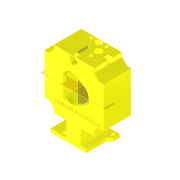
# Autodesk Inventor part: 20_Cube_Insert_Autofocus_KES400a_mirrorinsert
Saved by Autodesk Inventor 2022 (Build 260153000, 153)
## iProperties
Created: 2019-07-01
Part Number: 20_Cube_Insert_Autofocus_KES400a_mirrorinsert
Material: Generic
Document SubType Name: Modeling
Designer: diederichbenedict
Density: 1 g/cm^3
Appearance: Glatt - Gelb
Author: diederichbenedict
Autodesk Inventor part; units mm, degrees
ref_plane "YZ Plane" through (0, 0, 0) normal (1, 0, 0) x (0, 1, 0)
ref_plane "XZ Plane" through (0, 0, 0) normal (0, 1, 0) x (-1, 0, 0)
ref_plane "Work Plane1" through (-56.3599, 0, 22) normal (0, 0, -1) x (-1, 0, 0)
sketch "Sketch1" plane through (-56.3599, 0, 22) normal (0, 0, -1) x (-1, 0, 0)
  line L0 (-4.0299, -0.3538) -> (-2.2322, 1.4439) construction
  arc A0 (-1.4439, 2.2322) -> (-2.2322, 1.4439) centre (-0.9299, 0.9299) ccw construction
  line L1 (-1.4439, 2.2322) -> (0.3538, 4.0299) construction
  line L2 (-37.8299, 42.8299) -> (-37.8299, 37.8299) construction
  line L3 (-37.8299, 37.8299) -> (-42.9208, 37.8299) construction
  line L4 (-37.8299, 42.2137) -> (-37.8299, 45.8299) construction
  line L5 (-37.8299, 45.8299) -> (-4.0299, 45.8299) construction
  line L6 (-4.0299, 45.8299) -> (-4.0299, 42.2137) construction
  line L7 (-4.0299, 4.0299) -> (0.3538, 4.0299) projected
  circle A1 centre (-20.9299, 20.9299) radius 17.5 projected
  line L8 (-20.9299, 58.9723) -> (17.1124, 20.9299) construction
  line L9 (17.1124, 20.9299) -> (-20.9299, -17.1124) construction
  line L10 (-20.9299, -17.1124) -> (-58.9723, 20.9299) construction
  line L11 (-58.9723, 20.9299) -> (-20.9299, 58.9723) construction
  line L12 (-20.9299, 58.9723) -> (-20.9299, -17.1124) construction
  line L13 (17.1124, 20.9299) -> (-58.9723, 20.9299) construction
  line L14 (-20.9299, 58.9723) -> (32.8701, 58.9723) construction
  line L15 (-43.4299, 43.4299) -> (1.5701, 43.4299) construction
  line L16 (1.5701, 43.4299) -> (1.5701, -1.5701) construction
  line L17 (1.5701, -1.5701) -> (-43.4299, -1.5701) construction
  line L18 (-43.4299, -1.5701) -> (-43.4299, 43.4299) construction
  line L19 (-43.4299, 43.4299) -> (1.5701, -1.5701) construction
  line L20 (1.5701, 43.4299) -> (-43.4299, -1.5701) construction
  line L21 (-43.4299, 5.3876) -> (-43.4299, 36.4723)
  line L22 (-43.4299, 36.4723) -> (-36.4723, 43.4299)
  line L23 (-36.4723, 43.4299) -> (-5.3876, 43.4299)
  line L24 (-5.3876, 43.4299) -> (1.5701, 36.4723)
  line L25 (1.5701, 36.4723) -> (1.5701, 5.3876)
  line L26 (1.5701, 5.3876) -> (-5.3876, -1.5701)
  line L27 (-5.3876, -1.5701) -> (-36.4723, -1.5701)
  line L28 (-36.4723, -1.5701) -> (-43.4299, 5.3876)
  line L29 (-4.0299, 42.2137) -> (-37.8299, 42.2137) projected
  line L30 (-4.0299, -0.3538) -> (-4.0299, 4.0299) projected
  circle A2 centre (-20.9299, 20.9299) radius 1.5
  line L31 (-10.9299, 10.9299) -> (-30.9299, 10.9299) construction
  line L32 (-30.9299, 10.9299) -> (-30.9299, 30.9299) construction
  line L33 (-30.9299, 30.9299) -> (-10.9299, 30.9299) construction
  line L34 (-10.9299, 30.9299) -> (-10.9299, 10.9299) construction
  line L35 (-10.9299, 10.9299) -> (-30.9299, 30.9299) construction
  line L36 (-30.9299, 10.9299) -> (-10.9299, 30.9299) construction
  circle A3 centre (-30.9299, 30.9299) radius 1.4
  circle A4 centre (-30.9299, 10.9299) radius 1.4
  circle A5 centre (-10.9299, 10.9299) radius 1.4
  line L37 (-45.8299, 37.8299) -> (-42.0723, 37.8299) construction
  line L38 (-42.1723, 37.7299) -> (-45.8299, 37.7299)
  line L39 (-45.8299, 37.7299) -> (-45.8299, 4.1299)
  line L40 (-45.8299, 4.1299) -> (-42.1723, 4.1299)
  line L41 (-42.1723, 4.1299) -> (-42.1723, 37.7299)
  line L42 (-45.8299, 4.0299) -> (-42.0723, 4.0299) construction
  line L43 (-45.8299, 37.8299) -> (-42.0723, 37.8299) projected
  line L44 (-37.7299, 45.8299) -> (-4.1299, 45.8299)
  line L45 (-4.1299, 45.8299) -> (-4.1299, 42.1723)
  line L46 (-4.1299, 42.1723) -> (-37.7299, 42.1723)
  line L47 (-37.7299, 42.1723) -> (-37.7299, 45.8299)
  line L48 (0.4701, 37.8299) -> (0.4701, 4.0299) construction
  line L49 (0.4701, 4.0299) -> (3.9701, 4.0299) construction
  line L50 (3.9701, 37.8299) -> (3.9701, 4.0299) construction
  line L51 (0.4701, 37.8299) -> (3.9701, 37.8299) construction
  line L52 (-45.8299, -3.9701) -> (-4.0299, -3.9701) construction
  line L53 (0.3124, 37.7299) -> (3.9701, 37.7299)
  line L54 (3.9701, 37.7299) -> (3.9701, 4.1299)
  line L55 (3.9701, 4.1299) -> (0.3124, 4.1299)
  line L56 (0.3124, 4.1299) -> (0.3124, 37.7299)
  line L57 (-4.1299, -0.3538) -> (-37.7299, -0.3538)
  line L58 (-37.7299, -0.3538) -> (-37.7299, -3.9701)
  line L59 (-37.7299, -3.9701) -> (-4.1299, -3.9701)
  line L60 (-4.1299, -3.9701) -> (-4.1299, -0.3538)
  line L61 (-14.9299, -3.9701) -> (-26.9299, -3.9701)
  line L62 (-26.9299, -3.9701) -> (-26.9299, -15.9701)
  line L63 (-26.9299, -15.9701) -> (-14.9299, -15.9701)
  line L64 (-14.9299, -15.9701) -> (-14.9299, -3.9701)
  line L65 (-14.9299, -3.9701) -> (-26.9299, -15.9701) construction
  line L66 (-26.9299, -3.9701) -> (-14.9299, -15.9701) construction
  point P0 (-37.8299, 4.0299)
  point P1 (-20.9299, -9.9701)
  point P2 (-20.9299, -3.9701)
  point P3 (-14.9299, -3.9701)
  point P4 (-4.1713, -0.3538)
  point P5 (0.3124, 4.1299)
  point P6 (-42.1723, 4.1299)
  point P7 (-37.6885, -0.3538)
  point P8 (-26.9299, -3.9701)
  dimension "d18" = 53.8
  dimension "d19" = 45
  dimension "d20" = 53.8
  dimension "d21" = 45
  dimension "d22" = 45
  dimension "d30" = 20
  dimension "d31" = 20
  dimension "d32" = 2.8
  dimension "d33" = 2.8
  dimension "d34" = 2.8
  dimension "d35" = 3
  dimension "d36" = 0.1
  dimension "d37" = 0.1
  dimension "d38" = 0.1
  dimension "d39" = 0.1
  dimension "d196" = 12
  dimension "d197" = 12
  constraints: 98 end point, 22 point on line, 16 parallel, 11 midpoint, 9 perpendicular, 8 horizontal, 4 centre point, 4 coincident, 1 equal length
  measures "d18" distance of L8.start L8.end
  measures "d19" angle of L8 L14
  measures "d20" distance of L8.end L9.end
  measures "d21" distance of L16.end L17.end
  measures "d22" distance of L15.end L16.end
  measures "d30" distance of L32.end L33.end
  measures "d31" distance of L31.end L32.end
  measures "d32" diameter of A3
  measures "d33" diameter of A4
  measures "d34" diameter of A5
  measures "d35" diameter of A2
  measures "d36" distance between parallel lines of L38 L43
  measures "d37" distance between parallel lines of L40 L42
  measures "d38" distance between parallel lines of L45 L6
  measures "d39" distance between parallel lines of L4 L47
  measures "d196" distance of L63.end L62.end
  measures "d197" distance of L62.end L61.end
extrude "Extrusion1" add sketch "Sketch1" along normal blind 24 contours L30 L26 L57 L28 L41 L22 L46 L24 L56 L7 | L7 L26 L30 | L56 L24 L25 L26 | L26 L25 L24 L53 L54 L55 | L57 L60 L59 L58 L28 L27 L26 | L26 L27 L28 L57 | L46 L22 L29 L24 | L24 L29 L45 | L40 L39 L38 L22 L21 L28 | L28 L21 L22 L41 | L29 L22 L23 L24 | L24 L23 L22 L29 L47 L44 L45 | L47 L29 L22 | L64 L63 L62 L59 | A1 | A2 | A3 | A4 | A5
sketch "Skizze4" plane through (-56.3599, 0, -2) normal (0, 0, -1) x (-1, 0, 0)
  line L0 (-37.7299, 42.1723) -> (-42.1723, 37.7299) projected
  line L1 (-42.1723, 37.7299) -> (-45.8299, 37.7299) projected
  line L2 (-45.8299, 37.7299) -> (-45.8299, 4.1299) construction
  line L3 (-45.8299, 4.1299) -> (-42.1723, 4.1299) projected
  line L4 (-42.1723, 4.1299) -> (-37.6885, -0.3538) projected
  line L5 (-37.6885, -0.3538) -> (-37.7299, -0.3538) projected
  line L6 (-37.7299, -0.3538) -> (-37.7299, -3.9701) projected
  line L7 (-37.7299, -3.9701) -> (-26.9299, -3.9701) construction
  line L8 (-4.1299, -3.9701) -> (-4.1299, -0.3538) projected
  line L9 (-4.1713, -0.3538) -> (0.3124, 4.1299) projected
  line L10 (0.3124, 4.1299) -> (3.9701, 4.1299) projected
  line L11 (3.9701, 4.1299) -> (3.9701, 37.7299) construction
  line L12 (3.9701, 37.7299) -> (0.3124, 37.7299) projected
  line L13 (0.3124, 37.7299) -> (-4.1299, 42.1723) projected
  line L14 (-4.1299, 42.1723) -> (-4.1299, 45.8299) projected
  line L15 (-4.1299, 45.8299) -> (-37.7299, 45.8299) construction
  line L16 (-37.7299, 45.8299) -> (-37.7299, 42.1723) projected
  line L17 (-37.9299, 46.0299) -> (-3.9299, 46.0299) construction
  line L18 (-3.9299, 46.0299) -> (-3.9299, 42.2551)
  line L19 (-3.9299, 42.2551) -> (0.3953, 37.9299)
  line L20 (0.3953, 37.9299) -> (4.1701, 37.9299)
  line L21 (4.1701, 37.9299) -> (4.1701, 3.9299) construction
  line L22 (4.1701, 3.9299) -> (0.3953, 3.9299)
  line L23 (0.3953, 3.9299) -> (-3.9299, -0.3953)
  line L24 (-3.9299, -0.3953) -> (-3.9299, -4.1701)
  line L25 (-3.9299, -4.1701) -> (-37.9299, -4.1701) construction
  line L26 (-37.9299, -4.1701) -> (-37.9299, -0.3953)
  line L27 (-37.9299, -0.3953) -> (-42.2551, 3.9299)
  line L28 (-42.2551, 3.9299) -> (-46.0299, 3.9299)
  line L29 (-46.0299, 3.9299) -> (-46.0299, 37.9299) construction
  line L30 (-46.0299, 37.9299) -> (-42.2551, 37.9299)
  line L31 (-42.2551, 37.9299) -> (-37.9299, 42.2551)
  line L32 (-37.9299, 42.2551) -> (-37.9299, 46.0299)
  line L33 (-45.8299, 37.7299) -> (-45.8299, 37.9299)
  line L34 (-4.1299, 45.8299) -> (-37.7299, 45.8299) projected
  line L35 (-37.7299, 45.8299) -> (-37.9299, 45.8299)
  line L36 (-4.1299, 45.8299) -> (-3.9299, 45.8299)
  line L37 (3.9701, 37.7299) -> (3.9701, 37.9299)
  line L38 (3.9701, 4.1299) -> (3.9701, 37.7299) projected
  line L39 (3.9701, 4.1299) -> (3.9701, 3.9299)
  line L40 (-4.1299, -3.9701) -> (-3.9299, -3.9701)
  line L41 (-37.7299, -3.9701) -> (-37.9299, -3.9701)
  line L42 (-45.8299, 4.1299) -> (-45.8299, 3.9299)
  line L43 (-4.1299, -0.3538) -> (-4.1713, -0.3538) projected
  line L44 (-14.9299, -15.9701) -> (-14.9299, -3.9701) projected
  line L45 (-14.9299, -3.9701) -> (-4.1299, -3.9701) projected
  line L46 (-26.9299, -3.9701) -> (-26.9299, -15.9701) projected
  line L47 (-26.9299, -15.9701) -> (-14.9299, -15.9701) projected
  point P0 (-56.3599, 0)
  dimension "d40" = 0.2
  constraints: 48 end point, 12 point on line, 4 perpendicular, 15 other
  measures "d40" distance between parallel lines of L15 L17
extrude "IM_offset" add sketch "Skizze4" against normal up to surface (24 mm away)
ref_plane "Arbeitsebene5" through (-35.4299, 3.9299, 22) normal (-1, 0, 0) x (0, 0, 1)
ref_plane "Arbeitsebene6" through (-18.4299, 20.9299, 22) normal (0, 1, 0) x (-1, 0, 0)
chamfer "Fase2" distance 0.5 angle 45 34 edges at (-35.4299, 45.8299, 22) (-18.4299, 44.0425, 22) (-16.2673, 40.0925, 22) (-12.3173, 37.9299, 22) (-10.5299, 20.9299, 22) (-12.3173, 3.9299, 22) (-16.2673, 1.7673, 22) (-18.4299, -2.1827, 22) (-46.9299, -3.9701, 22) (-23.9299, -3.9701, 22) (-52.4299, -2.1827, 22) (-54.5925, 1.7673, 22) (-58.5425, 3.9299, 22) (-60.3299, 20.9299, 22) (-58.5425, 37.9299, 22) (-54.5925, 40.0925, 22) (-54.5925, 1.7673, -2) (-58.5425, 3.9299, -2) (-60.3299, 20.9299, -2) (-52.4299, -2.1827, -2) (-46.9299, -3.9701, -2) (-23.9299, -3.9701, -2) (-18.4299, -2.1827, -2) (-16.2673, 1.7673, -2) (-12.3173, 3.9299, -2) (-10.5299, 20.9299, -2) (-12.3173, 37.9299, -2) (-16.2673, 40.0925, -2) (-18.4299, 44.0425, -2) (-35.4299, 45.8299, -2) (-52.4299, 44.0425, -2) (-54.5925, 40.0925, -2) (-58.5425, 37.9299, -2) (-52.4299, 44.0425, 22)
sketch "Skizze32" plane through (-56.3599, 0, 22) normal (0, 0, 1) x (1, 0, 0)
  line L0 (4.6074, 8.4523) -> (68.202, 8.4523) construction
  line L1 (68.202, 8.4523) -> (68.202, -1.1922) construction
  line L2 (68.202, -1.1922) -> (4.6074, -1.1922) construction
  line L3 (4.6074, -1.1922) -> (4.6074, 8.4523) construction
  line L4 (7.5956, 5.2466) -> (6.6687, 5.2466)
  line L5 (6.6687, 5.2466) -> (5.8407, 6.4848)
  line L6 (5.8407, 6.4848) -> (5.69, 6.2772)
  line L7 (5.69, 6.2772) -> (5.69, 5.2466)
  line L8 (5.69, 5.2466) -> (4.9237, 5.2466)
  line L9 (4.9237, 5.2466) -> (4.9237, 8.2966)
  line L10 (4.9237, 8.2966) -> (5.69, 8.2966)
  line L11 (5.69, 8.2966) -> (5.69, 6.9347)
  line L12 (5.69, 6.9347) -> (6.6687, 8.2966)
  line L13 (6.6687, 8.2966) -> (7.5511, 8.2966)
  line L14 (7.5511, 8.2966) -> (6.4636, 6.8803)
  line L15 (6.4636, 6.8803) -> (7.5956, 5.2466)
  line L16 (7.8452, 5.2466) -> (7.8452, 8.2966)
  line L17 (7.8452, 8.2966) -> (9.9066, 8.2966)
  line L18 (9.9066, 8.2966) -> (9.9066, 7.7157)
  line L19 (9.9066, 7.7157) -> (8.6065, 7.7157)
  line L20 (8.6065, 7.7157) -> (8.6065, 7.1794)
  line L21 (8.6065, 7.1794) -> (9.8052, 7.1794)
  line L22 (9.8052, 7.1794) -> (9.8052, 6.5985)
  line L23 (9.8052, 6.5985) -> (8.6065, 6.5985)
  line L24 (8.6065, 6.5985) -> (8.6065, 5.8274)
  line L25 (8.6065, 5.8274) -> (9.9066, 5.8274)
  line L26 (9.9066, 5.8274) -> (9.9066, 5.2466)
  line L27 (9.9066, 5.2466) -> (7.8452, 5.2466)
  spline S0 degree 2 poles (11.3673, 5.1922) (11.0163, 5.1922) (10.4874, 5.3281) (10.26, 5.427) knots 0 0 0 1 2 2 2
  line L28 (10.26, 5.427) -> (10.26, 6.1536)
  line L29 (10.26, 6.1536) -> (10.3292, 6.1536)
  spline S1 degree 2 poles (10.3292, 6.1536) (10.5591, 5.9584) (11.1103, 5.7483) (11.3698, 5.7483) knots 0 0 0 1 2 2 2
  spline S2 degree 2 poles (11.3698, 5.7483) (11.4365, 5.7483) (11.6515, 5.778) (11.7158, 5.8076) knots 0 0 0 1 2 2 2
  spline S3 degree 2 poles (11.7158, 5.8076) (11.7949, 5.8422) (11.9061, 5.9683) (11.9061, 6.0696) knots 0 0 0 1 2 2 2
  spline S4 degree 2 poles (11.9061, 6.0696) (11.9061, 6.1858) (11.7257, 6.3291) (11.6021, 6.3613) knots 0 0 0 1 2 2 2
  spline S5 degree 2 poles (11.6021, 6.3613) (11.4464, 6.4033) (11.093, 6.475) (10.9372, 6.5293) knots 0 0 0 1 2 2 2
  spline S6 degree 2 poles (10.9372, 6.5293) (10.5838, 6.6529) (10.2773, 7.0756) (10.2773, 7.3919) knots 0 0 0 1 2 2 2
  spline S7 degree 2 poles (10.2773, 7.3919) (10.2773, 7.8195) (11.0015, 8.3509) (11.5453, 8.3509) knots 0 0 0 1 2 2 2
  spline S8 degree 2 poles (11.5453, 8.3509) (11.8171, 8.3509) (12.356, 8.2397) (12.5685, 8.1458) knots 0 0 0 1 2 2 2
  line L30 (12.5685, 8.1458) -> (12.5685, 7.4488)
  line L31 (12.5685, 7.4488) -> (12.5018, 7.4488)
  spline S9 degree 2 poles (12.5018, 7.4488) (12.3312, 7.5946) (11.8419, 7.7948) (11.5848, 7.7948) knots 0 0 0 1 2 2 2
  spline S10 degree 2 poles (11.5848, 7.7948) (11.4835, 7.7948) (11.3253, 7.7652) (11.2363, 7.7256) knots 0 0 0 1 2 2 2
  spline S11 degree 2 poles (11.2363, 7.7256) (11.1646, 7.6935) (11.0608, 7.5649) (11.0608, 7.4859) knots 0 0 0 1 2 2 2
  spline S12 degree 2 poles (11.0608, 7.4859) (11.0608, 7.3672) (11.2264, 7.2313) (11.4637, 7.1769) knots 0 0 0 1 2 2 2
  spline S13 degree 2 poles (11.4637, 7.1769) (11.6169, 7.1423) (11.9012, 7.0756) (12.0643, 7.0187) knots 0 0 0 1 2 2 2
  spline S14 degree 2 poles (12.0643, 7.0187) (12.3807, 6.9025) (12.6896, 6.517) (12.6896, 6.2006) knots 0 0 0 1 2 2 2
  spline S15 degree 2 poles (12.6896, 6.2006) (12.6896, 5.7458) (11.9753, 5.1922) (11.3673, 5.1922) knots 0 0 0 1 2 2 2
  line L32 (15.3541, 5.9584) -> (14.9413, 5.9584)
  line L33 (14.9413, 5.9584) -> (14.9413, 5.2391)
  line L34 (14.9413, 5.2391) -> (14.2023, 5.2391)
  line L35 (14.2023, 5.2391) -> (14.2023, 5.9584)
  line L36 (14.2023, 5.9584) -> (12.8577, 5.9584)
  line L37 (12.8577, 5.9584) -> (12.8577, 6.5269)
  line L38 (12.8577, 6.5269) -> (14.1776, 8.2966)
  line L39 (14.1776, 8.2966) -> (14.9413, 8.2966)
  line L40 (14.9413, 8.2966) -> (14.9413, 6.5071)
  line L41 (14.9413, 6.5071) -> (15.3541, 6.5071)
  line L42 (15.3541, 6.5071) -> (15.3541, 5.9584)
  line L43 (14.2023, 6.5071) -> (14.2023, 7.5452)
  line L44 (14.2023, 7.5452) -> (13.4287, 6.5071)
  line L45 (13.4287, 6.5071) -> (14.2023, 6.5071)
  spline S16 degree 2 poles (17.9493, 6.7716) (17.9493, 6.3761) (17.8232, 5.7829) (17.6823, 5.5827) knots 0 0 0 1 2 2 2
  spline S17 degree 2 poles (17.6823, 5.5827) (17.5439, 5.385) (17.0966, 5.1823) (16.7752, 5.1823) knots 0 0 0 1 2 2 2
  spline S18 degree 2 poles (16.7752, 5.1823) (16.4515, 5.1823) (16.0066, 5.385) (15.8657, 5.5876) knots 0 0 0 1 2 2 2
  spline S19 degree 2 poles (15.8657, 5.5876) (15.7248, 5.7878) (15.5987, 6.3761) (15.5987, 6.7716) knots 0 0 0 1 2 2 2
  spline S20 degree 2 poles (15.5987, 6.7716) (15.5987, 7.1769) (15.7248, 7.7503) (15.8682, 7.9579) knots 0 0 0 1 2 2 2
  spline S21 degree 2 poles (15.8682, 7.9579) (16.0115, 8.1606) (16.4638, 8.3583) (16.7752, 8.3583) knots 0 0 0 1 2 2 2
  spline S22 degree 2 poles (16.7752, 8.3583) (17.104, 8.3583) (17.5439, 8.1507) (17.6848, 7.9456) knots 0 0 0 1 2 2 2
  spline S23 degree 2 poles (17.6848, 7.9456) (17.8232, 7.7454) (17.9493, 7.1547) (17.9493, 6.7716) knots 0 0 0 1 2 2 2
  spline S24 degree 2 poles (17.1806, 6.7716) (17.1806, 7.3376) (16.9952, 7.7948) (16.7752, 7.7948) knots 0 0 0 1 2 2 2
  spline S25 degree 2 poles (16.7752, 7.7948) (16.5553, 7.7948) (16.3674, 7.3376) (16.3674, 6.7691) knots 0 0 0 1 2 2 2
  spline S26 degree 2 poles (16.3674, 6.7691) (16.3674, 6.2105) (16.5553, 5.7458) (16.7752, 5.7458) knots 0 0 0 1 2 2 2
  spline S27 degree 2 poles (16.7752, 5.7458) (16.9928, 5.7458) (17.1806, 6.2105) (17.1806, 6.7716) knots 0 0 0 1 2 2 2
  spline S28 degree 2 poles (20.6211, 6.7716) (20.6211, 6.3761) (20.4951, 5.7829) (20.3542, 5.5827) knots 0 0 0 1 2 2 2
  spline S29 degree 2 poles (20.3542, 5.5827) (20.2158, 5.385) (19.7684, 5.1823) (19.4471, 5.1823) knots 0 0 0 1 2 2 2
  spline S30 degree 2 poles (19.4471, 5.1823) (19.1233, 5.1823) (18.6784, 5.385) (18.5375, 5.5876) knots 0 0 0 1 2 2 2
  spline S31 degree 2 poles (18.5375, 5.5876) (18.3966, 5.7878) (18.2706, 6.3761) (18.2706, 6.7716) knots 0 0 0 1 2 2 2
  spline S32 degree 2 poles (18.2706, 6.7716) (18.2706, 7.1769) (18.3966, 7.7503) (18.54, 7.9579) knots 0 0 0 1 2 2 2
  spline S33 degree 2 poles (18.54, 7.9579) (18.6834, 8.1606) (19.1357, 8.3583) (19.4471, 8.3583) knots 0 0 0 1 2 2 2
  spline S34 degree 2 poles (19.4471, 8.3583) (19.7758, 8.3583) (20.2158, 8.1507) (20.3566, 7.9456) knots 0 0 0 1 2 2 2
  spline S35 degree 2 poles (20.3566, 7.9456) (20.4951, 7.7454) (20.6211, 7.1547) (20.6211, 6.7716) knots 0 0 0 1 2 2 2
  spline S36 degree 2 poles (19.8524, 6.7716) (19.8524, 7.3376) (19.6671, 7.7948) (19.4471, 7.7948) knots 0 0 0 1 2 2 2
  spline S37 degree 2 poles (19.4471, 7.7948) (19.2271, 7.7948) (19.0393, 7.3376) (19.0393, 6.7691) knots 0 0 0 1 2 2 2
  spline S38 degree 2 poles (19.0393, 6.7691) (19.0393, 6.2105) (19.2271, 5.7458) (19.4471, 5.7458) knots 0 0 0 1 2 2 2
  spline S39 degree 2 poles (19.4471, 5.7458) (19.6646, 5.7458) (19.8524, 6.2105) (19.8524, 6.7716) knots 0 0 0 1 2 2 2
  line L46 (21.9978, 5.2466) -> (23.0285, 8.2966)
  line L47 (23.0285, 8.2966) -> (23.8639, 8.2966)
  line L48 (23.8639, 8.2966) -> (24.8946, 5.2466)
  line L49 (24.8946, 5.2466) -> (24.1061, 5.2466)
  line L50 (24.1061, 5.2466) -> (23.9158, 5.8694)
  line L51 (23.9158, 5.8694) -> (22.9568, 5.8694)
  line L52 (22.9568, 5.8694) -> (22.764, 5.2466)
  line L53 (22.764, 5.2466) -> (21.9978, 5.2466)
  line L54 (23.7477, 6.4231) -> (23.4363, 7.4315)
  line L55 (23.4363, 7.4315) -> (23.1224, 6.4231)
  line L56 (23.1224, 6.4231) -> (23.7477, 6.4231)
  line L57 (27.2921, 5.2466) -> (26.5753, 5.2466)
  line L58 (26.5753, 5.2466) -> (26.5753, 5.5011)
  spline S40 degree 2 poles (26.5753, 5.5011) (26.3899, 5.3454) (26.0785, 5.1823) (25.8635, 5.1823) knots 0 0 0 1 2 2 2
  spline S41 degree 2 poles (25.8635, 5.1823) (25.5224, 5.1823) (25.1393, 5.6148) (25.1393, 6.0498) knots 0 0 0 1 2 2 2
  line L59 (25.1393, 6.0498) -> (25.1393, 7.5476)
  line L60 (25.1393, 7.5476) -> (25.861, 7.5476)
  line L61 (25.861, 7.5476) -> (25.861, 6.4058)
  spline S42 degree 2 poles (25.861, 6.4058) (25.861, 6.2278) (25.8783, 6.0004) (25.9129, 5.9238) knots 0 0 0 1 2 2 2
  spline S43 degree 2 poles (25.9129, 5.9238) (25.9475, 5.8521) (26.0834, 5.778) (26.207, 5.778) knots 0 0 0 1 2 2 2
  spline S44 degree 2 poles (26.207, 5.778) (26.2812, 5.778) (26.4888, 5.8521) (26.5753, 5.9164) knots 0 0 0 1 2 2 2
  line L62 (26.5753, 5.9164) -> (26.5753, 7.5476)
  line L63 (26.5753, 7.5476) -> (27.2921, 7.5476)
  line L64 (27.2921, 7.5476) -> (27.2921, 5.2466)
  spline S45 degree 2 poles (28.7207, 5.2021) (28.2832, 5.2021) (27.8828, 5.5629) (27.8828, 5.9732) knots 0 0 0 1 2 2 2
  line L65 (27.8828, 5.9732) -> (27.8828, 7.0484)
  line L66 (27.8828, 7.0484) -> (27.6084, 7.0484)
  line L67 (27.6084, 7.0484) -> (27.6084, 7.5476)
  line L68 (27.6084, 7.5476) -> (27.8828, 7.5476)
  line L69 (27.8828, 7.5476) -> (27.8828, 8.2051)
  line L70 (27.8828, 8.2051) -> (28.5996, 8.2051)
  line L71 (28.5996, 8.2051) -> (28.5996, 7.5476)
  line L72 (28.5996, 7.5476) -> (29.2916, 7.5476)
  line L73 (29.2916, 7.5476) -> (29.2916, 7.0484)
  line L74 (29.2916, 7.0484) -> (28.5996, 7.0484)
  line L75 (28.5996, 7.0484) -> (28.5996, 6.2303)
  spline S46 degree 2 poles (28.5996, 6.2303) (28.5996, 6.1092) (28.6045, 5.9287) (28.6342, 5.857) knots 0 0 0 1 2 2 2
  spline S47 degree 2 poles (28.6342, 5.857) (28.6638, 5.7854) (28.8096, 5.7013) (28.9481, 5.7013) knots 0 0 0 1 2 2 2
  spline S48 degree 2 poles (28.9481, 5.7013) (29.0074, 5.7013) (29.1928, 5.7508) (29.2298, 5.7705) knots 0 0 0 1 2 2 2
  line L76 (29.2298, 5.7705) -> (29.2916, 5.7705)
  line L77 (29.2916, 5.7705) -> (29.2916, 5.2663)
  spline S49 degree 2 poles (29.2916, 5.2663) (29.1754, 5.2367) (28.9135, 5.2021) (28.7207, 5.2021) knots 0 0 0 1 2 2 2
  spline S50 degree 2 poles (31.7904, 6.3959) (31.7904, 5.8274) (31.1701, 5.1749) (30.6041, 5.1749) knots 0 0 0 1 2 2 2
  spline S51 degree 2 poles (30.6041, 5.1749) (30.0405, 5.1749) (29.4152, 5.8274) (29.4152, 6.3959) knots 0 0 0 1 2 2 2
  spline S52 degree 2 poles (29.4152, 6.3959) (29.4152, 6.9693) (30.0405, 7.6193) (30.6041, 7.6193) knots 0 0 0 1 2 2 2
  spline S53 degree 2 poles (30.6041, 7.6193) (31.1676, 7.6193) (31.7904, 6.9668) (31.7904, 6.3959) knots 0 0 0 1 2 2 2
  spline S54 degree 2 poles (31.0564, 6.3909) (31.0564, 6.5961) (30.9896, 6.8704) (30.9303, 6.952) knots 0 0 0 1 2 2 2
  spline S55 degree 2 poles (30.9303, 6.952) (30.866, 7.0385) (30.7054, 7.1052) (30.6041, 7.1052) knots 0 0 0 1 2 2 2
  spline S56 degree 2 poles (30.6041, 7.1052) (30.5052, 7.1052) (30.3495, 7.0459) (30.2852, 6.9619) knots 0 0 0 1 2 2 2
  spline S57 degree 2 poles (30.2852, 6.9619) (30.2234, 6.8828) (30.1493, 6.6035) (30.1493, 6.3909) knots 0 0 0 1 2 2 2
  spline S58 degree 2 poles (30.1493, 6.3909) (30.1493, 6.1808) (30.2185, 5.9213) (30.2753, 5.8422) knots 0 0 0 1 2 2 2
  spline S59 degree 2 poles (30.2753, 5.8422) (30.3322, 5.7631) (30.5052, 5.689) (30.609, 5.689) knots 0 0 0 1 2 2 2
  spline S60 degree 2 poles (30.609, 5.689) (30.6955, 5.689) (30.8735, 5.7631) (30.9278, 5.8373) knots 0 0 0 1 2 2 2
  spline S61 degree 2 poles (30.9278, 5.8373) (30.9896, 5.9238) (31.0564, 6.1734) (31.0564, 6.3909) knots 0 0 0 1 2 2 2
  line L78 (33.6417, 7.8912) -> (33.5873, 7.8912)
  spline S62 degree 2 poles (33.5873, 7.8912) (33.5453, 7.9036) (33.3698, 7.9431) (33.2932, 7.9431) knots 0 0 0 1 2 2 2
  spline S63 degree 2 poles (33.2932, 7.9431) (33.0757, 7.9431) (32.9175, 7.7849) (32.9175, 7.5649) knots 0 0 0 1 2 2 2
  line L79 (32.9175, 7.5649) -> (32.9175, 7.5476)
  line L80 (32.9175, 7.5476) -> (33.4885, 7.5476)
  line L81 (33.4885, 7.5476) -> (33.4885, 7.0484)
  line L82 (33.4885, 7.0484) -> (32.9422, 7.0484)
  line L83 (32.9422, 7.0484) -> (32.9422, 5.2466)
  line L84 (32.9422, 5.2466) -> (32.2254, 5.2466)
  line L85 (32.2254, 5.2466) -> (32.2254, 7.0484)
  line L86 (32.2254, 7.0484) -> (31.9387, 7.0484)
  line L87 (31.9387, 7.0484) -> (31.9387, 7.5476)
  line L88 (31.9387, 7.5476) -> (32.2254, 7.5476)
  line L89 (32.2254, 7.5476) -> (32.2254, 7.6119)
  spline S64 degree 2 poles (32.2254, 7.6119) (32.2254, 8.0321) (32.6679, 8.4523) (33.1177, 8.4523) knots 0 0 0 1 2 2 2
  spline S65 degree 2 poles (33.1177, 8.4523) (33.2734, 8.4523) (33.5428, 8.43) (33.6417, 8.4102) knots 0 0 0 1 2 2 2
  line L90 (33.6417, 8.4102) -> (33.6417, 7.8912)
  spline S66 degree 2 poles (35.9823, 6.3959) (35.9823, 5.8274) (35.362, 5.1749) (34.796, 5.1749) knots 0 0 0 1 2 2 2
  spline S67 degree 2 poles (34.796, 5.1749) (34.2324, 5.1749) (33.6071, 5.8274) (33.6071, 6.3959) knots 0 0 0 1 2 2 2
  spline S68 degree 2 poles (33.6071, 6.3959) (33.6071, 6.9693) (34.2324, 7.6193) (34.796, 7.6193) knots 0 0 0 1 2 2 2
  spline S69 degree 2 poles (34.796, 7.6193) (35.3595, 7.6193) (35.9823, 6.9668) (35.9823, 6.3959) knots 0 0 0 1 2 2 2
  spline S70 degree 2 poles (35.2483, 6.3909) (35.2483, 6.5961) (35.1815, 6.8704) (35.1222, 6.952) knots 0 0 0 1 2 2 2
  spline S71 degree 2 poles (35.1222, 6.952) (35.0579, 7.0385) (34.8973, 7.1052) (34.796, 7.1052) knots 0 0 0 1 2 2 2
  spline S72 degree 2 poles (34.796, 7.1052) (34.6971, 7.1052) (34.5414, 7.0459) (34.4771, 6.9619) knots 0 0 0 1 2 2 2
  spline S73 degree 2 poles (34.4771, 6.9619) (34.4153, 6.8828) (34.3412, 6.6035) (34.3412, 6.3909) knots 0 0 0 1 2 2 2
  spline S74 degree 2 poles (34.3412, 6.3909) (34.3412, 6.1808) (34.4104, 5.9213) (34.4672, 5.8422) knots 0 0 0 1 2 2 2
  spline S75 degree 2 poles (34.4672, 5.8422) (34.5241, 5.7631) (34.6971, 5.689) (34.8009, 5.689) knots 0 0 0 1 2 2 2
  spline S76 degree 2 poles (34.8009, 5.689) (34.8874, 5.689) (35.0654, 5.7631) (35.1197, 5.8373) knots 0 0 0 1 2 2 2
  spline S77 degree 2 poles (35.1197, 5.8373) (35.1815, 5.9238) (35.2483, 6.1734) (35.2483, 6.3909) knots 0 0 0 1 2 2 2
  spline S78 degree 2 poles (37.49, 5.1848) (37.2058, 5.1848) (36.7337, 5.3281) (36.5582, 5.4764) knots 0 0 0 1 2 2 2
  spline S79 degree 2 poles (36.5582, 5.4764) (36.3877, 5.6272) (36.1949, 6.0795) (36.1949, 6.386) knots 0 0 0 1 2 2 2
  spline S80 degree 2 poles (36.1949, 6.386) (36.1949, 6.7172) (36.4025, 7.1794) (36.5829, 7.3277) knots 0 0 0 1 2 2 2
  spline S81 degree 2 poles (36.5829, 7.3277) (36.7535, 7.471) (37.2182, 7.6094) (37.4703, 7.6094) knots 0 0 0 1 2 2 2
  spline S82 degree 2 poles (37.4703, 7.6094) (37.6606, 7.6094) (38.0412, 7.5205) (38.234, 7.4241) knots 0 0 0 1 2 2 2
  line L91 (38.234, 7.4241) -> (38.234, 6.8111)
  line L92 (38.234, 6.8111) -> (38.1425, 6.8111)
  spline S83 degree 2 poles (38.1425, 6.8111) (38.0981, 6.8531) (37.9745, 6.952) (37.9003, 6.9915) knots 0 0 0 1 2 2 2
  spline S84 degree 2 poles (37.9003, 6.9915) (37.8212, 7.036) (37.626, 7.0953) (37.5049, 7.0953) knots 0 0 0 1 2 2 2
  spline S85 degree 2 poles (37.5049, 7.0953) (37.2305, 7.0953) (36.929, 6.7122) (36.929, 6.386) knots 0 0 0 1 2 2 2
  spline S86 degree 2 poles (36.929, 6.386) (36.929, 6.0399) (37.2503, 5.6989) (37.5172, 5.6989) knots 0 0 0 1 2 2 2
  spline S87 degree 2 poles (37.5172, 5.6989) (37.6532, 5.6989) (37.8558, 5.7607) (37.93, 5.8051) knots 0 0 0 1 2 2 2
  spline S88 degree 2 poles (37.93, 5.8051) (38.0017, 5.8472) (38.1055, 5.9411) (38.1425, 5.9782) knots 0 0 0 1 2 2 2
  line L93 (38.1425, 5.9782) -> (38.234, 5.9782)
  line L94 (38.234, 5.9782) -> (38.234, 5.3627)
  spline S89 degree 2 poles (38.234, 5.3627) (38.1722, 5.3355) (38.0116, 5.2663) (37.9275, 5.2441) knots 0 0 0 1 2 2 2
  spline S90 degree 2 poles (37.9275, 5.2441) (37.8237, 5.2144) (37.6408, 5.1848) (37.49, 5.1848) knots 0 0 0 1 2 2 2
  line L95 (40.7106, 5.2466) -> (39.9938, 5.2466)
  line L96 (39.9938, 5.2466) -> (39.9938, 5.5011)
  spline S91 degree 2 poles (39.9938, 5.5011) (39.8084, 5.3454) (39.497, 5.1823) (39.282, 5.1823) knots 0 0 0 1 2 2 2
  spline S92 degree 2 poles (39.282, 5.1823) (38.9409, 5.1823) (38.5578, 5.6148) (38.5578, 6.0498) knots 0 0 0 1 2 2 2
  line L97 (38.5578, 6.0498) -> (38.5578, 7.5476)
  line L98 (38.5578, 7.5476) -> (39.2795, 7.5476)
  line L99 (39.2795, 7.5476) -> (39.2795, 6.4058)
  spline S93 degree 2 poles (39.2795, 6.4058) (39.2795, 6.2278) (39.2968, 6.0004) (39.3314, 5.9238) knots 0 0 0 1 2 2 2
  spline S94 degree 2 poles (39.3314, 5.9238) (39.366, 5.8521) (39.5019, 5.778) (39.6255, 5.778) knots 0 0 0 1 2 2 2
  spline S95 degree 2 poles (39.6255, 5.778) (39.6997, 5.778) (39.9073, 5.8521) (39.9938, 5.9164) knots 0 0 0 1 2 2 2
  line L100 (39.9938, 5.9164) -> (39.9938, 7.5476)
  line L101 (39.9938, 7.5476) -> (40.7106, 7.5476)
  line L102 (40.7106, 7.5476) -> (40.7106, 5.2466)
  spline S96 degree 2 poles (41.9588, 5.1848) (41.7066, 5.1848) (41.2543, 5.296) (41.106, 5.3701) knots 0 0 0 1 2 2 2
  line L103 (41.106, 5.3701) -> (41.106, 5.9757)
  line L104 (41.106, 5.9757) -> (41.1654, 5.9757)
  spline S97 degree 2 poles (41.1654, 5.9757) (41.2173, 5.9361) (41.3483, 5.8422) (41.4644, 5.7903) knots 0 0 0 1 2 2 2
  spline S98 degree 2 poles (41.4644, 5.7903) (41.5658, 5.7434) (41.8154, 5.6766) (41.9637, 5.6766) knots 0 0 0 1 2 2 2
  spline S99 degree 2 poles (41.9637, 5.6766) (42.1145, 5.6766) (42.3468, 5.7705) (42.3468, 5.8719) knots 0 0 0 1 2 2 2
  spline S100 degree 2 poles (42.3468, 5.8719) (42.3468, 5.951) (42.2405, 6.035) (42.0873, 6.0696) knots 0 0 0 1 2 2 2
  spline S101 degree 2 poles (42.0873, 6.0696) (42.0057, 6.0919) (41.7561, 6.1388) (41.6597, 6.1685) knots 0 0 0 1 2 2 2
  spline S102 degree 2 poles (41.6597, 6.1685) (41.3878, 6.2525) (41.1159, 6.5812) (41.1159, 6.8506) knots 0 0 0 1 2 2 2
  spline S103 degree 2 poles (41.1159, 6.8506) (41.1159, 7.0039) (41.2568, 7.2758) (41.3952, 7.382) knots 0 0 0 1 2 2 2
  spline S104 degree 2 poles (41.3952, 7.382) (41.5312, 7.4859) (41.934, 7.6094) (42.1886, 7.6094) knots 0 0 0 1 2 2 2
  spline S105 degree 2 poles (42.1886, 7.6094) (42.4308, 7.6094) (42.8362, 7.513) (42.9746, 7.4463) knots 0 0 0 1 2 2 2
  line L105 (42.9746, 7.4463) -> (42.9746, 6.863)
  line L106 (42.9746, 6.863) -> (42.9178, 6.863)
  spline S106 degree 2 poles (42.9178, 6.863) (42.8807, 6.8927) (42.72, 6.9891) (42.6459, 7.0237) knots 0 0 0 1 2 2 2
  spline S107 degree 2 poles (42.6459, 7.0237) (42.5544, 7.0632) (42.332, 7.1176) (42.2158, 7.1176) knots 0 0 0 1 2 2 2
  spline S108 degree 2 poles (42.2158, 7.1176) (42.0601, 7.1176) (41.8451, 7.0113) (41.8451, 6.9248) knots 0 0 0 1 2 2 2
  spline S109 degree 2 poles (41.8451, 6.9248) (41.8451, 6.8457) (41.9513, 6.7567) (42.1293, 6.7122) knots 0 0 0 1 2 2 2
  spline S110 degree 2 poles (42.1293, 6.7122) (42.2207, 6.69) (42.4605, 6.648) (42.5717, 6.6109) knots 0 0 0 1 2 2 2
  spline S111 degree 2 poles (42.5717, 6.6109) (42.8189, 6.5318) (43.0759, 6.2228) (43.0759, 5.9658) knots 0 0 0 1 2 2 2
  spline S112 degree 2 poles (43.0759, 5.9658) (43.0759, 5.8051) (42.9252, 5.511) (42.7843, 5.4122) knots 0 0 0 1 2 2 2
  spline S113 degree 2 poles (42.7843, 5.4122) (42.6385, 5.3034) (42.2381, 5.1848) (41.9588, 5.1848) knots 0 0 0 1 2 2 2
  point P0 (56.3599, 0)
  constraints: 2 other
extrude "Extrusion27" cut sketch "Skizze32" against normal blind 1
sketch "Skizze33" plane through (-56.3599, 0, 22) normal (0, 0, 1) x (1, 0, 0)
  line L0 (37.4299, -3.4701) -> (26.9299, -3.4701) projected
  line L1 (37.4299, -0.1882) -> (37.4299, -3.4701) projected
  line L2 (42.048, 4.4299) -> (37.4299, -0.1882) projected
  line L3 (45.3299, 4.4299) -> (42.048, 4.4299) projected
  line L4 (45.3299, 37.4299) -> (45.3299, 4.4299) projected
  line L5 (42.048, 37.4299) -> (45.3299, 37.4299) projected
  line L6 (37.4299, 42.048) -> (42.048, 37.4299) projected
  line L7 (37.4299, 45.3299) -> (37.4299, 42.048) projected
  line L8 (4.4299, 45.3299) -> (37.4299, 45.3299) projected
  line L9 (4.4299, 42.048) -> (4.4299, 45.3299) projected
  line L10 (-0.1882, 37.4299) -> (4.4299, 42.048) projected
  line L11 (-3.4701, 37.4299) -> (-0.1882, 37.4299) projected
  line L12 (-3.4701, 4.4299) -> (-3.4701, 37.4299) projected
  line L13 (-0.1882, 4.4299) -> (-3.4701, 4.4299) projected
  line L14 (4.4299, -0.1882) -> (-0.1882, 4.4299) projected
  line L15 (4.4299, -3.4701) -> (4.4299, -0.1882) projected
  line L16 (26.3918, 7.9579) -> (26.3918, 8.3583) projected
  line L17 (16.7752, 2.6565) -> (17.6848, 2.6565) projected
  line L18 (25.5638, 5.5827) -> (25.5638, 5.1823) projected
  line L19 (16.7752, 1.0351) -> (15.8657, 1.0351) projected
  line L20 (14.9413, 8.2966) -> (14.9413, 6.5071) projected
  line L21 (14.2023, 5.9584) -> (12.8577, 5.9584) projected
  line L22 (14.2023, 5.2391) -> (14.2023, 5.9584) projected
  line L23 (14.9413, 5.2391) -> (14.2023, 5.2391) projected
  line L24 (14.9413, 5.9584) -> (14.9413, 5.2391) projected
  line L25 (15.3541, 5.9584) -> (14.9413, 5.9584) projected
  line L26 (15.3541, 6.5071) -> (15.3541, 5.9584) projected
  line L27 (14.9413, 6.5071) -> (15.3541, 6.5071) projected
  line L28 (7.8452, 8.2966) -> (9.9066, 8.2966) projected
  line L29 (7.8452, 5.2466) -> (7.8452, 8.2966) projected
  line L30 (8.6065, 6.5985) -> (8.6065, 5.8274) projected
  line L31 (9.8052, 6.5985) -> (8.6065, 6.5985) projected
  line L32 (9.9066, 8.2966) -> (9.9066, 7.7157) projected
  line L33 (6.6687, 8.2966) -> (7.5511, 8.2966) projected
  line L34 (7.5511, 8.2966) -> (6.4636, 6.8803) projected
  line L35 (6.4636, 6.8803) -> (7.5956, 5.2466) projected
  line L36 (7.5956, 5.2466) -> (6.6687, 5.2466) projected
  line L37 (6.6687, 5.2466) -> (5.8407, 6.4848) projected
  line L38 (5.8407, 6.4848) -> (5.69, 6.2772) projected
  line L39 (5.69, 6.2772) -> (5.69, 5.2466) projected
  line L40 (5.69, 5.2466) -> (4.9237, 5.2466) projected
  line L41 (4.9237, 5.2466) -> (4.9237, 8.2966) projected
  line L42 (4.9237, 8.2966) -> (5.69, 8.2966) projected
  line L43 (5.69, 8.2966) -> (5.69, 6.9347) projected
  line L44 (5.69, 6.9347) -> (6.6687, 8.2966) projected
  line L45 (10.26, 5.427) -> (10.26, 6.1536) projected
  line L46 (10.2773, 2.3723) -> (11.5453, 2.3723) projected
  line L47 (15.7959, 8.3509) -> (15.7959, 8.1458) projected
  line L48 (12.5685, 8.1458) -> (12.5685, 7.4488) projected
  line L49 (12.5685, 7.4488) -> (12.5018, 7.4488) projected
  line L50 (12.5018, 3.5092) -> (11.5848, 3.5092) projected
  line L51 (16.52, 7.7948) -> (16.52, 7.7256) projected
  line L52 (14.2023, 6.5071) -> (14.2023, 7.5452) projected
  line L53 (14.2023, 7.5452) -> (13.4287, 6.5071) projected
  line L54 (28.7472, 5.7458) -> (28.7472, 6.7716) projected
  line L55 (30.4255, 5.7458) -> (30.4255, 6.7716) projected
  line L56 (23.1224, 6.4231) -> (23.7477, 6.4231) projected
  circle A0 centre (20.9299, 20.9299) radius 24.4
  circle A1 centre (20.9299, 20.9299) radius 10
  line L57 (37.9299, 45.8299) -> (3.9299, 45.8299) projected
  line L58 (14.9299, -15.9701) -> (14.9299, -3.4701) projected
  line L59 (26.9299, -15.9701) -> (14.9299, -15.9701) projected
  line L60 (26.9299, -3.4701) -> (26.9299, -15.9701) projected
  line L61 (14.9299, -3.4701) -> (4.4299, -3.4701) projected
  line L62 (12.8577, 5.9584) -> (12.8577, 6.5269) projected
  line L63 (12.8577, 6.5269) -> (14.1776, 8.2966) projected
  line L64 (14.1776, 8.2966) -> (14.9413, 8.2966) projected
  line L65 (28.9299, 14.0017) -> (22.9299, 10.5376)
  line L66 (10.9299, 17.4658) -> (10.9299, 24.394)
  line L67 (22.9299, 31.3222) -> (28.9299, 27.8581)
  arc A2 (22.9299, 31.3222) -> (10.9299, 24.394) centre (18.9299, 24.394) ccw
  arc A3 (28.9299, 14.0017) -> (28.9299, 27.8581) centre (24.9299, 20.9299) ccw
  arc A4 (10.9299, 17.4658) -> (22.9299, 10.5376) centre (18.9299, 17.4658) ccw
  point P0 (56.3599, 0)
  point P1 (16.7752, 8.3583)
  point P2 (16.7752, 5.1823)
  point P3 (11.5453, 8.3509)
  point P4 (11.5848, 7.7948)
  point P5 (-0.5475, 33.3299)
  point P6 (42.4074, 33.3299)
  point P7 (20.9299, -3.8701)
  point P8 (40.9299, 20.9299)
  point P9 (10.9299, 3.6094)
  point P10 (10.9299, 38.2504)
  point P11 (25.9299, 12.2697)
  point P12 (10.9299, 20.9299)
  point P13 (25.9299, 29.5902)
  dimension "d189" = 20
  dimension "d213" = 8
  constraints: 10 tangent, 6 end point, 6 horizontal alignment, 6 point on circle, 6 point on line, 5 centre point, 3 coincident, 3 vertical alignment, 2 equal radius, 35 other
  measures "d189" diameter of A1
  measures "d213" radius of A2
extrude "Extrusion28" cut sketch "Skizze33" against normal through all contours A1 | A1 L67 A3 L65 | A1 L66 A2 L67 | L65 A4 L66 A1
chamfer "Fase3" distance 1 angle 45 6 edges at (-41.4299, 31.3222, 22) (-30.4299, 29.5902, 22) (-23.4299, 20.9299, 22) (-30.4299, 12.2697, 22) (-41.4299, 10.5376, 22) (-45.4299, 20.9299, 22)
sketch "Skizze34" plane through (-41.4299, -15.9701, 22) normal (0, -1, 0) x (1, 0, 0)
  line L0 (12, 0) -> (0, 0) projected
  line L1 (0, 0) -> (0, -24) projected
  line L2 (12, -24) -> (0, -24) projected
  line L3 (12, 0) -> (12, -24) projected
  circle A0 centre (6, -17) radius 3.5
  point P0 (41.4299, -22)
  dimension "d198" = 7
  dimension "d199" = 7
  constraints: 1 centre point
  measures "d198" diameter of A0
  measures "d199" distance from line of A0.centre L2
extrude "Extrusion29" cut sketch "Skizze34" against normal blind 50 contours A0
sketch "Skizze35" plane through (-41.4299, -15.9701, 22) normal (0, -1, 0) x (1, 0, 0)
  arc A0 (-10.1555, -25.7) -> (-9.1555, -24.7) centre (-10.1555, -24.7) ccw construction
  line L0 (-10.1555, -25.7) -> (-13.3, -25.7) construction
  line L1 (-13.3, -25.7) -> (-13.3, 0) construction
  line L2 (-13.3, 0) -> (-3.7723, 0) construction
  arc A1 (-2.7723, -1) -> (-3.7723, 0) centre (-3.7723, -1) ccw construction
  line L3 (-2.7723, -1) -> (-2.7723, -2.8624) construction
  arc A2 (-2.7723, -2.8624) -> (-1.7723, -3.8624) centre (-1.7723, -2.8624) ccw construction
  line L4 (-1.7723, -3.8624) -> (16.7, -3.8624) construction
  line L5 (16.7, -3.8624) -> (16.7, -15.397) construction
  arc A3 (16.7, -15.397) -> (17.7, -16.397) centre (17.7, -15.397) ccw construction
  line L6 (17.7, -16.397) -> (18.7, -16.397) construction
  arc A4 (19.7, -17.397) -> (18.7, -16.397) centre (18.7, -17.397) ccw construction
  line L7 (19.7, -17.397) -> (19.7, -19.9624) construction
  arc A5 (18.7, -20.9624) -> (19.7, -19.9624) centre (18.7, -19.9624) ccw construction
  line L8 (18.7, -20.9624) -> (-8.1555, -20.9624) construction
  arc A6 (-8.1555, -20.9624) -> (-9.1555, -21.9624) centre (-8.1555, -21.9624) ccw construction
  line L9 (-9.1555, -21.9624) -> (-9.1555, -24.7) construction
  line L10 (-0.8, -19) -> (14.7, -19) construction
  line L11 (14.7, -19) -> (14.7, -5.5) construction
  line L12 (14.7, -5.5) -> (-0.8, -5.5) construction
  line L13 (-0.8, -5.5) -> (-0.8, -19) construction
  circle A7 centre (-10.8, -23) radius 1 construction
  circle A8 centre (-4.3, -2.5) radius 1 construction
  circle A9 centre (17.2, -18) radius 1 construction
  circle A10 centre (-4.3, -2.5) radius 1.6
  circle A11 centre (-10.8, -23) radius 1.6
  circle A12 centre (17.2, -18) radius 1.6
  circle A13 centre (6, -13) radius 3.4826 projected
  line L14 (-7.8964, -25.7) -> (-7.8964, -20.9624)
  line L15 (-7.8964, -20.9624) -> (19.7, -20.9624)
  line L16 (19.7, -20.9624) -> (19.7, -15.397)
  line L17 (19.7, -15.397) -> (16.7, -15.397)
  line L18 (16.7, -15.397) -> (16.7, -3.8624)
  line L19 (16.7, -3.8624) -> (-3.7723, 0)
  line L20 (-8.2612, 0) -> (-8.2612, -1) projected
  line L21 (-8.2612, 0) -> (-13.3, 0)
  line L22 (-15.1181, 0) -> (-10.5, 0) projected
  line L23 (-13.3, 0) -> (-13.3, -25.7)
  line L24 (-7.8964, -25.7) -> (-13.3, -25.7)
  line L25 (-3.7723, 0) -> (-8.2612, 0)
  line L26 (-3.7723, 0) -> (16.7, 0)
  line L27 (16.7, 0) -> (16.7, -3.8624)
  circle A14 centre (6, -17) radius 3.5 projected
  circle A15 centre (-4.3, -6.5) radius 1.6
  circle A16 centre (-10.8, -27) radius 1.6
  circle A17 centre (17.2, -22) radius 1.6
  line L28 (-7.8964, -29.7) -> (-7.8964, -24.9624)
  line L29 (-7.8964, -24.9624) -> (19.7, -24.9624)
  line L30 (19.7, -24.9624) -> (19.7, -19.397)
  line L31 (19.7, -19.397) -> (16.7, -19.397)
  line L32 (16.7, -19.397) -> (16.7, -7.8624)
  line L33 (16.7, -7.8624) -> (-3.7723, -4)
  line L34 (-8.2612, -4) -> (-13.3, -4)
  line L35 (-13.3, -4) -> (-13.3, -29.7)
  line L36 (-7.8964, -29.7) -> (-13.3, -29.7)
  line L37 (-3.7723, -4) -> (-8.2612, -4)
  line L38 (-3.7723, -4) -> (16.7, -4)
  line L39 (16.7, -4) -> (16.7, -7.8624)
  circle A18 centre (-4.3, -6.5) radius 1.6
  circle A19 centre (-10.8, -27) radius 1.6
  circle A20 centre (17.2, -22) radius 1.6
  line L40 (-7.8964, -29.7) -> (-7.8964, -24.9624)
  line L41 (-7.8964, -24.9624) -> (19.7, -24.9624)
  line L42 (19.7, -24.9624) -> (19.7, -19.397)
  line L43 (19.7, -19.397) -> (16.7, -19.397)
  line L44 (16.7, -19.397) -> (16.7, -7.8624)
  line L45 (16.7, -7.8624) -> (-3.7723, -4)
  line L46 (-8.2612, -4) -> (-13.3, -4)
  line L47 (-13.3, -4) -> (-13.3, -29.7)
  line L48 (-7.8964, -29.7) -> (-13.3, -29.7)
  line L49 (-3.7723, -4) -> (-8.2612, -4)
  line L50 (-3.7723, -4) -> (16.7, -4)
  line L51 (16.7, -4) -> (16.7, -7.8624)
  point P0 (41.4299, -22)
  point P1 (16.7, -3.8624)
  point P2 (19.7, -20.9624)
  point P3 (-13.3, -25.7)
  point P4 (-7.8964, -25.7)
  point P5 (-7.8964, -24.9624)
  dimension "d202" = 3.2
  dimension "d203" = 3.2
  dimension "d204" = 3.2
  dimension "d238" = 3.2
  dimension "d239" = 3.2
  dimension "d240" = 3.2
  dimension "d241" = 3.2
  dimension "d242" = 3.2
  dimension "d243" = 3.2
  constraints: 72 end point, 9 centre point, 9 perpendicular, 6 collinear, 4 point on line, 3 coincident, 3 horizontal, 3 vertical, 1 point on circle
  measures "d202" diameter of A10
  measures "d203" diameter of A11
  measures "d204" diameter of A12
  measures "d238" diameter of A15
  measures "d239" diameter of A16
  measures "d240" diameter of A17
  measures "d241" diameter of A18
  measures "d242" diameter of A19
  measures "d243" diameter of A20
extrude "Extrusion30" add sketch "Skizze35" along normal blind 3 contours A10 L37 L34 L23 L21 L25 L19 L18 L38 | A10 L33 L18 L32 A12 L31 L16 L15 A17 L14 L24 A16 L23 L34 L37 | L38 L18 L33 | L19 L26 L27 | L24 A16 L28 L36 L35 | L32 L31 A12 | L30 L29 L14 L15 A17 | A11 | A13 A14 picked at (16.5852, -17.506) picked at (5.8772, -10.8663)
sketch "Skizze37" plane through (-56.3599, 0, -2) normal (0, 0, -1) x (-1, 0, 0)
  line L0 (-24.4299, -18.9701) -> (-24.4299, 11.4036) projected
  line L1 (-17.4299, -18.9701) -> (-17.4299, 9.6077) projected
  line L2 (-68.4258, 20.9299) -> (16.0361, 20.9299) projected
  line L3 (-20.9299, 58.1899) -> (-20.9299, -28.3301) projected
  line L4 (-7.4299, 7.4299) -> (-34.4299, 7.4299)
  line L5 (-34.4299, 7.4299) -> (-34.4299, 34.4299)
  line L6 (-34.4299, 34.4299) -> (-7.4299, 34.4299)
  line L7 (-7.4299, 34.4299) -> (-7.4299, 7.4299)
  line L8 (-7.4299, 7.4299) -> (-34.4299, 34.4299) construction
  line L9 (-34.4299, 7.4299) -> (-7.4299, 34.4299) construction
  point P0 (-56.3599, 0)
  point P1 (-20.9299, 20.9299)
  dimension "d214" = 27
  dimension "d215" = 27
  constraints: 12 end point, 2 midpoint, 2 parallel, 2 point on line, 1 horizontal, 1 perpendicular
  measures "d214" distance between parallel lines of L6 L4
  measures "d215" distance between parallel lines of L7 L5
extrude "Extrusion32" cut sketch "Skizze37" against normal blind 20
sketch "Skizze38" plane through (-52.4299, 45.8299, -1.5) normal (0, 1, 0) x (1, 0, 0)
  line L0 (0, 0) -> (34, 0) projected
  line L1 (0, 0) -> (0, -23) projected
  line L2 (34, -23) -> (0, -23) projected
  line L3 (34, 0) -> (34, -23) projected
  line L4 (33.5, 0.5) -> (0.5, 0.5) projected
  circle A0 centre (17, -6.5) radius 3.5 projected
  line L5 (23.5, -15.5) -> (10.5, -15.5)
  line L6 (10.5, -15.5) -> (10.5, -2.5)
  line L7 (10.5, -2.5) -> (23.5, -2.5)
  line L8 (23.5, -2.5) -> (23.5, -15.5)
  line L9 (23.5, -15.5) -> (10.5, -2.5) construction
  line L10 (10.5, -15.5) -> (23.5, -2.5) construction
  line L11 (0.5, -23.5) -> (33.5, -23.5) projected
  circle A1 centre (10.5, -2.5) radius 1.4
  circle A2 centre (23.5, -2.5) radius 1.4
  circle A3 centre (23.5, -15.5) radius 1.4
  circle A4 centre (17, -2.5) radius 3
  circle A5 centre (23.5, -9) radius 3
  point P0 (52.4299, -1.5)
  point P1 (17, -9)
  dimension "d226" = 13
  dimension "d227" = 13
  dimension "d228" = 24
  dimension "d229" = 3
  dimension "d230" = 2.8
  dimension "d231" = 2.8
  dimension "d232" = 2.8
  dimension "d233" = 6
  dimension "d234" = 6
  constraints: 12 end point, 5 centre point, 4 midpoint, 3 coincident, 2 parallel, 1 horizontal, 1 perpendicular
  measures "d226" distance of L6.end L7.end
  measures "d227" distance of L5.end L6.end
  measures "d228" distance between parallel lines of L11 L4
  measures "d229" distance between parallel lines of L7 L4
  measures "d230" diameter of A1
  measures "d231" diameter of A2
  measures "d232" diameter of A3
  measures "d233" diameter of A4
  measures "d234" diameter of A5
extrude "Extrusion33" cut sketch "Skizze38" against normal blind 16 contours A4 L0 | L0 A4 L7 | L7 A4 A0 | A1 L6 L7 | L7 L6 A1 | A0 A4 | A2 L8 L7 | L7 L8 A2 | A5 L8 | L8 A5 | A3 L8 L5 | L5 L8 A3 picked at (16.8879, -3.8427)
chamfer "Fase4" distance 3 angle 45 2 edges at (-49.3263, -17.4701, -2.9624) (-24.7299, -17.4701, 2.603)
sketch "Skizze39" plane through (-18.4299, 42.2551, -1.5) normal (1, 0, 0) x (0, 0, -1)
  line L0 (-12, 3.5748) -> (-12, -7.8252) projected
  line L1 (-6, 3.5748) -> (-6, -7.8252) projected
  line L2 (0, 0) -> (-23, 0) projected
  circle A0 centre (-9, 0) radius 3
  circle A1 centre (-9, 1.225) radius 0.9
  point P0 (-1.5, -42.2551)
  dimension "d245" = 1.8
  constraints: 2 centre point, 2 tangent, 1 point on line
  measures "d245" diameter of A1
hole "Bohrung2" at (-18.4299, 43.4801, 7.5) direction (-1, 0, 0) diameter 2.8 end through all counterbore diameter 6.5 counterbore depth 4
sketch "Skizze40" plane through (-56.3599, 0, 22) normal (0, 0, 1) x (1, 0, 0)
  line L0 (24.4299, 45.8299) -> (24.4299, 34.4299) projected
  line L1 (17.9299, 45.8299) -> (17.9299, 34.4299) projected
  line L2 (20.9299, 45.3299) -> (20.9299, 34.4299) projected
  circle A0 centre (20.9299, 42.9846) radius 1.4
  point P0 (56.3599, 0)
  dimension "d253" = 2.8
  constraints: 1 centre point, 1 point on line
  measures "d253" diameter of A0
hole "Bohrung3" at (-35.4299, 42.9846, 22) direction (0, 0, -1) diameter 2.8 end through all counterbore diameter 6.5 counterbore depth 4
body "Solid1"
